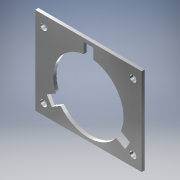
# Autodesk Inventor part: shaft_holder
Saved by Autodesk Inventor 2018 (Build 220112000, 112)
## iProperties
Created: 2018-04-03
Part Number: shaft_holder
Material: アルミニウム 6061
Document SubType Name: Modeling
Designer: NaMACHAN
Density: 2.7 g/cm^3
Appearance: アルミニウム - フラット
Author: NaMACHAN
Autodesk Inventor part; units mm, degrees
ref_plane "YZ Plane" through (0, 0, 0) normal (1, 0, 0) x (0, 1, 0)
ref_plane "XZ Plane" through (0, 0, 0) normal (0, 1, 0) x (-1, 0, 0)
ref_plane "XY Plane" through (0, 0, 0) normal (0, 0, 1) x (1, 0, 0)
sketch "スケッチ1" plane through (0, 0, 0) normal (0, 1, 0) x (-1, 0, 0)
  line L0 (25, 23) -> (-25, 23)
  line L1 (-25, 23) -> (-25, -16.9)
  line L2 (-25, -16.9) -> (25, -16.9)
  line L3 (25, -16.9) -> (25, 23)
  circle A0 centre (0, 0) radius 16.5
  point P0 (0, 23)
  dimension "d0" = 50
  dimension "d1" = 16.9
  dimension "d2" = 23
  dimension "d3" = 33
  constraints: 8 end point, 2 parallel, 1 centre point, 1 coincident, 1 horizontal, 1 midpoint, 1 perpendicular, 1 vertical alignment
  measures "d0" distance of L1.end L2.end
  measures "d1" distance from line of point (0, 0) L2
  measures "d2" distance from line of L0 point (0, 0)
  measures "d3" diameter of A0
extrude "押し出し1" add sketch "スケッチ1" along normal blind 1.5
sketch "スケッチ2" plane through (0, 1.5, 0) normal (0, 1, 0) x (1, 0, 0)
  line L0 (-11.6489, 9.3236) -> (-17.278, 12.5736)
  line L1 (-17.278, 12.5736) -> (-19.528, 8.6764)
  line L2 (-19.528, 8.6764) -> (-13.8989, 5.4264)
  line L3 (-13.8989, 5.4264) -> (-11.6489, 9.3236)
  line L4 (-11.6489, 9.3236) -> (-19.528, 8.6764) construction
  line L5 (-17.278, 12.5736) -> (-13.8989, 5.4264) construction
  line L6 (19.528, 8.6764) -> (13.8989, 5.4264)
  line L7 (13.8989, 5.4264) -> (11.6489, 9.3236)
  line L8 (11.6489, 9.3236) -> (17.278, 12.5736)
  line L9 (17.278, 12.5736) -> (19.528, 8.6764)
  line L10 (19.528, 8.6764) -> (11.6489, 9.3236) construction
  line L11 (13.8989, 5.4264) -> (17.278, 12.5736) construction
  line L12 (-2.25, -21.25) -> (-2.25, -14.75)
  line L13 (-2.25, -14.75) -> (2.25, -14.75)
  line L14 (2.25, -14.75) -> (2.25, -21.25)
  line L15 (2.25, -21.25) -> (-2.25, -21.25)
  line L16 (-2.25, -21.25) -> (2.25, -14.75) construction
  line L17 (-2.25, -14.75) -> (2.25, -21.25) construction
  line L18 (25, 16.9) -> (-25, 16.9) projected
  point P0 (0, 0)
  point P1 (0, -18)
  point P2 (-15.5885, 9)
  point P3 (15.5885, 9)
  dimension "d6" = 120
  dimension "d7" = 120
  dimension "d8" = 18
  dimension "d9" = 18
  dimension "d10" = 18
  dimension "d11" = 30
  dimension "d12" = 30
  dimension "d13" = 4.5
  dimension "d14" = 6.5
  dimension "d15" = 4.5
  dimension "d16" = 6.5
  dimension "d17" = 4.5
  dimension "d18" = 6.5
  constraints: 36 end point, 6 midpoint, 6 parallel, 3 perpendicular, 1 horizontal, 1 vertical alignment
  measures "d8" distance of point (-15.588, 9) point (0, 0)
  measures "d9" distance of point (15.588, 9) point (0, 0)
  measures "d10" distance of point (0, -18) point (0, 0)
  measures "d11" angle of L18 L0
  measures "d12" angle of L18 L8
  measures "d13" distance of L6.end L7.end
  measures "d14" distance of L7.end L8.end
  measures "d15" distance of L2.end L0.start
  measures "d16" distance of L0.start L0.end
  measures "d17" distance of L12.end L13.end
  measures "d18" distance of L12.start L12.end
extrude "押し出し2" cut sketch "スケッチ2" against normal blind 1.5
sketch "スケッチ3" plane through (0, 1.5, 0) normal (0, 1, 0) x (1, 0, 0)
  line L0 (25, -23) -> (25, 16.9) projected
  line L1 (-25, -23) -> (25, -23) projected
  line L2 (-25, 16.9) -> (-25, -23) projected
  line L3 (25, 16.9) -> (-25, 16.9) projected
  point P0 (0, 0)
  point P1 (-21, -18)
  point P2 (-21, 2)
  point P3 (21, 2)
  point P4 (21, -18)
  dimension "d21" = 4
  dimension "d22" = 5
  dimension "d23" = 4
  dimension "d34" = 20
  constraints: 2 horizontal alignment, 2 vertical alignment
  measures "d21" distance from line of L0 point (21, -18)
  measures "d22" distance from line of L1 point (21, -18)
  measures "d23" distance from line of L2 point (-21, -18)
  measures "d34" distance of point (21, -18) point (21, 2)
hole "穴1" at (-21, 1.5, 18) at (-21, 1.5, -2) at (21, 1.5, -2) at (21, 1.5, 18) direction (0, -1, 0) diameter 3 end through all
